2.5mm bottom thin (Autodesk Fusion 360 design; units mm, degrees)
Autodesk Fusion 360 part; units mm, degrees
note: some values were not read from the file. Chosen so that the rebuilt part matches the saved one: which bodies a step acts on. Set by a fixed rule: which sketch regions a step uses.
sketch "Sketch1" plane through (0, 0, 0) normal (0, 0, 1) x (1, 0, 0)
  line L0 (-36.0939, 0.2498) -> (0, 0) construction
  line L1 (0, 0) -> (0.1129, 16.3059) construction
  line L2 (0.1129, 16.3059) -> (-35.9811, 16.5557) construction
  line L3 (-35.9811, 16.5557) -> (-36.0939, 0.2498) construction
  dimension "d1" = 3
  text T0 "2.5 mm bottom thin" font "Arial" height 3 align right bottom in box 36.0948 x 16.3063 at (-36.0939, 0.2498) x (0.999976, -0.006921) y (0.006921, 0.999976) spacing 1
  constraint coincident L0.end
extrude "Extrude1" add sketch "Sketch1" along normal blind 1 text T0 makes body 1 at (-28.1848, 1.2954, 0) makes body 2 at (-30.9414, 3.056, 0) makes body 3 at (-34.6225, 0.3576, 0) makes body 4 at (-13.1696, 1.328, 0) makes body 5 at (-15.1882, 1.1515, 0) makes body 6 at (-14.0238, 1.1435, 0) makes body 7 at (-24.6937, 1.2712, 0) makes body 8 at (-32.5906, 0.2256, 0.3333) makes body 9 at (-20.1638, 1.1396, 0.3333) makes body 10 at (-10.7172, 1.1745, 0) makes body 11 at (-1.761, 0.7366, 0.3333) makes body 12 at (-17.8291, 1.3602, 0) makes body 13 at (-5.0209, 1.0348, 0.3333) makes body 14 at (-2.3167, 1.4649, 0.3333) makes body 15 at (-2.6762, 2.7362, 0.3333) makes body 16 at (-5.8732, 1.0871, 0)
sketch "Sketch2" plane through (0, 0, 0) normal (0, 0, 1) x (1, 0, 0)
  line L0 (-33.8375, 4.0654) -> (-1.4845, 4.0654)
  line L1 (-1.4845, 4.0654) -> (-1.4845, -1.6678)
  line L2 (-1.4845, -1.6678) -> (-33.8375, -1.6678)
  line L3 (-33.8375, -1.6678) -> (-33.8375, 4.0654)
  circle A0 centre (-1.4845, 1.1988) radius 2.8666
  circle A1 centre (-33.8375, 1.1988) radius 2.8666
  constraint horizontal L0
  constraint vertical L1
  constraint horizontal L2
  constraint vertical L3
  constraint coincident L1.end A0
  constraint tangent L2 A0
  constraint coincident L0.end A0
  constraint coincident L2.end A1
  constraint tangent L2 A1
  constraint coincident L0.start A1
extrude "Extrude2" add sketch "Sketch2" against normal blind 1 bodies 1 2 3
